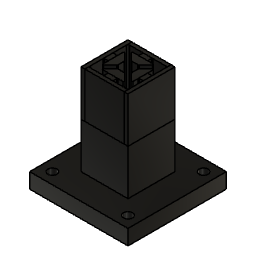
extrusion_hole (Autodesk Fusion 360 design; units mm, degrees)
Autodesk Fusion 360 part; units mm, degrees
note: some values were not read from the file. Chosen so that the rebuilt part matches the saved one: which bodies a step acts on.
sketch "Sketch1" plane through (0, 0, 0) normal (0, 0, 1) x (1, 0, 0)
  line L0 (15.5, -15.5) -> (-15.5, -15.5)
  line L1 (-15.5, -15.5) -> (-15.5, 15.5)
  line L2 (-15.5, 15.5) -> (15.5, 15.5)
  line L3 (15.5, 15.5) -> (15.5, -15.5)
  line L4 (15.5, -15.5) -> (-15.5, 15.5) construction
  line L5 (-15.5, -15.5) -> (15.5, 15.5) construction
  dimension "d11" = 31
  dimension "d12" = 31
  constraint horizontal L0
  constraint perpendicular L0 L1
  constraint parallel L0 L2
  constraint parallel L1 L3
  constraint coincident L4 origin
  constraint coincident L5 origin
  measures "d11" distance of L1.end L2.end
  measures "d12" distance of L0.end L1.end
extrude "Extrude1" add sketch "Sketch1" along normal blind 30 makes body 1
sketch "Sketch2" plane through (0, 0, 30) normal (0, 0, 1) x (-1, 0, 0)
  line L0 (-15.5, -15.5) -> (15.5, -15.5)
  line L1 (15.5, -15.5) -> (15.5, 15.5)
  line L2 (15.5, 15.5) -> (-15.5, 15.5)
  line L3 (-15.5, 15.5) -> (-15.5, -15.5)
  line L4 (-10.5, 3.5) -> (-12.5, 3.5)
  line L5 (10.5, 3.5) -> (10.5, 9.0858)
  line L6 (9.0858, -10.5) -> (2.5858, -4)
  line L7 (-12.5, -3.5) -> (-10.5, -3.5)
  line L8 (-10.5, 9.0858) -> (-10.5, 3.5)
  line L9 (9.0858, 10.5) -> (3.5, 10.5)
  line L10 (0, 0) -> (-4, 4) construction
  line L11 (-9.0858, -10.5) -> (-3.5, -10.5)
  line L12 (-9.0858, 10.5) -> (-2.5858, 4)
  line L13 (3.5, -12.5) -> (3.5, -10.5)
  line L14 (10.5, -3.5) -> (12.5, -3.5)
  line L15 (-2.5858, -4) -> (2.5858, -4)
  line L16 (-3.5, -10.5) -> (-3.5, -12.5)
  line L17 (2.5858, 4) -> (-2.5858, 4)
  line L18 (3.5, 10.5) -> (3.5, 12.5)
  line L19 (9.0858, 10.5) -> (2.5858, 4)
  line L20 (10.5, 9.0858) -> (4, 2.5858)
  line L21 (10.5, -9.0858) -> (4, -2.5858)
  line L22 (-10.5, -3.5) -> (-10.5, -9.0858)
  line L23 (-4, 2.5858) -> (-4, -2.5858)
  line L24 (3.5, -10.5) -> (9.0858, -10.5)
  line L25 (4, -2.5858) -> (4, 2.5858)
  line L26 (12.5, 3.5) -> (10.5, 3.5)
  line L27 (-3.5, -12.5) -> (-12.5, -12.5)
  line L28 (-12.5, 12.5) -> (-3.5, 12.5)
  line L29 (-10.5, -9.0858) -> (-4, -2.5858)
  line L30 (-9.0858, -10.5) -> (-2.5858, -4)
  line L31 (-3.5, 10.5) -> (-9.0858, 10.5)
  line L32 (-12.5, -12.5) -> (-12.5, -3.5)
  line L33 (12.5, -12.5) -> (3.5, -12.5)
  line L34 (10.5, -9.0858) -> (10.5, -3.5)
  line L35 (-12.5, 3.5) -> (-12.5, 12.5)
  line L36 (-3.5, 12.5) -> (-3.5, 10.5)
  line L37 (12.5, 12.5) -> (12.5, 3.5)
  line L38 (-10.5, 9.0858) -> (-4, 2.5858)
  line L39 (-4, -4) -> (0, 0) construction
  line L40 (3.5, 12.5) -> (12.5, 12.5)
  line L41 (12.5, -3.5) -> (12.5, -12.5)
  line L42 (10, 7.8787) -> (4.5, 2.3787)
  line L43 (4.5, -2.3787) -> (4.5, 2.3787)
  line L44 (10, -7.8787) -> (4.5, -2.3787)
  line L45 (10, -7.8787) -> (10, -3)
  line L46 (10, -3) -> (13, -3)
  line L47 (13, -3) -> (13, -13)
  line L48 (13, -13) -> (3, -13)
  line L49 (3, -13) -> (3, -10)
  line L50 (3, -10) -> (7.8787, -10)
  line L51 (7.8787, -10) -> (2.3787, -4.5)
  line L52 (-2.3787, -4.5) -> (2.3787, -4.5)
  line L53 (-7.8787, -10) -> (-2.3787, -4.5)
  line L54 (-7.8787, -10) -> (-3, -10)
  line L55 (-3, -10) -> (-3, -13)
  line L56 (-3, -13) -> (-13, -13)
  line L57 (-13, -13) -> (-13, -3)
  line L58 (-13, -3) -> (-10, -3)
  line L59 (-10, -3) -> (-10, -7.8787)
  line L60 (-10, -7.8787) -> (-4.5, -2.3787)
  line L61 (-4.5, 2.3787) -> (-4.5, -2.3787)
  line L62 (-10, 7.8787) -> (-4.5, 2.3787)
  line L63 (-10, 7.8787) -> (-10, 3)
  line L64 (-10, 3) -> (-13, 3)
  line L65 (-13, 3) -> (-13, 13)
  line L66 (-13, 13) -> (-3, 13)
  line L67 (-3, 13) -> (-3, 10)
  line L68 (-3, 10) -> (-7.8787, 10)
  line L69 (-7.8787, 10) -> (-2.3787, 4.5)
  line L70 (2.3787, 4.5) -> (-2.3787, 4.5)
  line L71 (7.8787, 10) -> (2.3787, 4.5)
  line L72 (7.8787, 10) -> (3, 10)
  line L73 (3, 10) -> (3, 13)
  line L74 (3, 13) -> (13, 13)
  line L75 (13, 13) -> (13, 3)
  line L76 (13, 3) -> (10, 3)
  line L77 (10, 3) -> (10, 7.8787)
  line L78 (4.5, -2.3787) -> (4.5, -4)
  line L79 (4.5, -4) -> (2.5858, -4)
  line L80 (4.5, -4) -> (5.3107, -3.1893)
  line L81 (10, -7.8787) -> (7.8787, -10)
  line L82 (10, -7.8787) -> (10, -10)
  line L83 (10, -10) -> (7.8787, -10)
  line L84 (4.5, -2.3787) -> (10, -2.3787)
  line L85 (10, -2.3787) -> (10, -7.8787)
  dimension "d16" = 360
  dimension "d17" = 8
  dimension "d18" = 2
  dimension "d19" = 2
  dimension "d20" = 2
  dimension "d21" = 9
  dimension "d22" = 9
  dimension "d23" = 135
  dimension "d24" = 8
  dimension "d25" = 0.5
  dimension "d32" = 9
  dimension "d33" = 9
  dimension "d34" = 1.1464
  dimension "d35" = 1.1464
  dimension "d36" = 2.1213
  dimension "d37" = 2.1213
  dimension "d38" = 3
  dimension "d39" = 4.7574
  dimension "d40" = 6
  dimension "d41" = 7.7782
  dimension "d42" = 5.5
  dimension "d43" = 5.5
  dimension "d44" = 5.5
  dimension "d45" = 10
  dimension "d46" = 12.5
  dimension "d47" = 2.5
  dimension "d48" = 31
  constraint horizontal L15
  constraint perpendicular L15 L25
  constraint parallel L15 L17
  constraint parallel L23 L25
  constraint coincident L10.start L39
  constraint coincident L39.end L10
  constraint coincident L10.start L39.end
  constraint perpendicular L13 L24
  constraint perpendicular L24 L34
  constraint parallel L6 L21
  constraint symmetric L6 L10 L21
  constraint perpendicular L15 L78
  constraint perpendicular L78 L79
  constraint coincident L44 L80.end
  constraint perpendicular L44 L80
  constraint perpendicular L51 L81
  constraint vertical L82
  constraint perpendicular L82 L83
  constraint perpendicular L45 L84
  constraint perpendicular L84 L85
  measures "d17" distance of L10.end L39.start
  measures "d18" distance of L6 L21
  measures "d19" distance of L14.start L14.end
  measures "d20" distance of L13.start L13.end
  measures "d21" distance of L13 L41
  measures "d22" distance of L14.end L33.start
  measures "d23" angle of L21 L25
  measures "d24" distance of L23 L25
  measures "d32" distance of L52 L70
  measures "d33" distance of L43 L61
  measures "d34" distance of L43.start L80
  measures "d35" distance of L78.end L80.end
  measures "d36" distance of L44.start L82.end
  measures "d37" distance of L50.end L82.end
  measures "d38" distance of L44.start L50.end
  measures "d39" distance of L42.end L43.start
  measures "d40" distance of L46 L76
  measures "d41" distance of L43.start L44.start
  measures "d42" distance of L43 L45.end
  measures "d43" distance of L44.start L84.end
  measures "d44" distance of L1 L85
  measures "d45" distance of L46 L48
  measures "d46" distance of L0 L46
  measures "d47" distance of L1 L47
  measures "d48" distance of L1 L3
extrude "Extrude2" add sketch "Sketch2" along normal blind 50 contours L0 L1 L2 L3 | L44 L45 L84 L85 bodies 1
fillet "Fillet1" radius 1 12 edges at (-13, 13, 55) (-4.5, 2.3787, 55) (-4.5, -2.3787, 55) (-13, -13, 55) (2.3787, -4.5, 55) (-2.3787, -4.5, 55) (-2.3787, 4.5, 55) (2.3787, 4.5, 55) (4.5, -2.3787, 55) (4.5, 2.3787, 55) (13, -13, 55) (13, 13, 55) on bodies 1
fillet "Fillet2" radius 0.5 24 edges at (-7.8787, 10, 55) (-10, 7.8787, 55) (-13, 3, 55) (-10, 3, 55) (-3, 10, 55) (-3, 13, 55) (3, 10, 55) (7.8787, 10, 55) (10, 7.8787, 55) (10, -7.8787, 55) (3, 13, 55) (10, 3, 55) (13, 3, 55) (10, -3, 55) (13, -3, 55) (7.8787, -10, 55) (3, -10, 55) (3, -13, 55) (-7.8787, -10, 55) (-10, -7.8787, 55) (-13, -3, 55) (-10, -3, 55) (-3, -10, 55) (-3, -13, 55) on bodies 1
extrude "Extrude3" cut 1 faces at (0.6548, 8.2857, 80) along direction (0, 0, -1) blind 20 on bodies 1 bodies 1
move_body "Move1" bodies 1 to x (1, 0, 0) y (0, 1, 0) z (0, 0, 1) at (0, 0, -30)
split "Split1" by plane through (0, 0, 0) normal (0, 0, 1) bodies 1 makes body 2 at (-15.5, -5.1667, 20)
split "Split2" by plane through (-13, 3, 0) normal (1, 0, 0) and through (13, 13, 0) normal (-1, 0, 0) bodies 2 makes body 3 at (-7.6953, -5.5739, 10) makes body 4 at (15.5, 5.1667, 20) makes body 5 at (4.3333, -15.5, 10) makes body 6 at (7.6953, 5.5739, 10) makes body 7 at (-4.3333, 15.5, 20)
split "Split3" by plane through (3, 13, 0) normal (0, -1, 0) and through (-3, 10, 0) normal (0, 1, 0) bodies 7 makes body 8 at (13, 12.3333, 10) makes body 9 at (-5.5739, 7.6953, 10) makes body 10 at (-12.9989, 12.0476, 10) makes body 11 at (3, 11.1667, 10)
split "Split4" by plane through (-3, -13, 0) normal (0, 1, 0) and through (3, -10, 0) normal (0, -1, 0) bodies 5 makes body 12 at (12.9989, -12.0476, 10) makes body 13 at (5.5739, -7.6953, 10) makes body 14 at (-13, -12.6667, 20) makes body 15 at (-3, -11.1667, 10)
split "Split5" by plane through (10, 3, 0) normal (1, 0, 0) bodies 6 makes body 16 at (13, 1.1667, 20)
split "Split6" by plane through (-10, -3, 0) normal (-1, 0, 0) bodies 3 makes body 17 at (-13, -1.1667, 20)
split "Split7" by plane through (3, 10, 0) normal (1, 0, 0) and through (-3, 13, 0) normal (-1, 0, 0) bodies 11 makes body 18 at (3.3333, 10, 10) makes body 19 at (3.4762, 12.9994, 10) makes body 20 at (-3.4762, 10.0006, 10) makes body 21 at (-3.0556, 12.7291, 10)
split "Split8" by plane through (-3, -10, 0) normal (-1, 0, 0) and through (3, -13, 0) normal (1, 0, 0) bodies 15 makes body 22 at (-3.4762, -10.0006, 10) makes body 23 at (-3.3333, -13, 10) makes body 24 at (3.0556, -10.2709, 10) makes body 25 at (3.4762, -12.9994, 10)
split "Split9" by plane through (10, -3, 0) normal (0, -1, 0) and through (13, 3, 0) normal (0, 1, 0) bodies 16 makes body 26 at (12.7291, -3.0556, 10) makes body 27 at (10.0006, -3.4762, 10) makes body 28 at (13, 3.1667, 10) makes body 29 at (10.2709, 3.0556, 10)
split "Split10" by plane through (-10, 3, 0) normal (0, 1, 0) and through (-13, -3, 0) normal (0, -1, 0) bodies 17 makes body 30 at (-10.2709, 3.0556, 10) makes body 31 at (-13, 3.1667, 20) makes body 32 at (-10.0006, -3.4762, 10) makes body 33 at (-12.7291, -3.0556, 10)
move_body "Move2" bodies 1 2 3 4 5 6 7 8 9 10 11 12 13 14 15 16 17 18 19 20 21 22 23 24 25 26 27 28 29 30 31 32 33 to x (1, 0, 0) y (0, 1, 0) z (0, 0, 1) at (0, 0, -30)
sketch "Sketch3" plane through (0, 0, -60) normal (0, 0, -1) x (1, 0, 0)
  line L0 (-15.5, -15.5) -> (15.5, -15.5)
  line L1 (15.5, -15.5) -> (15.5, 15.5)
  line L2 (15.5, 15.5) -> (-15.5, 15.5)
  line L3 (-15.5, 15.5) -> (-15.5, -15.5)
  line L4 (32.5, 32.5) -> (-32.5, 32.5)
  line L5 (-32.5, 32.5) -> (-32.5, -32.5)
  line L6 (-32.5, -32.5) -> (32.5, -32.5)
  line L7 (32.5, -32.5) -> (32.5, 32.5)
  line L8 (32.5, 32.5) -> (-32.5, -32.5) construction
  line L9 (-32.5, 32.5) -> (32.5, -32.5) construction
  circle A0 centre (25, 25) radius 3
  circle A1 centre (-25, 25) radius 3
  circle A2 centre (-25, -25) radius 3
  circle A3 centre (25, -25) radius 3
  dimension "d51" = 65
  dimension "d52" = 65
  dimension "d53" = 6
  dimension "d54" = 6
  dimension "d55" = 6
  dimension "d57" = 25
  dimension "d58" = 25
  dimension "d59" = 25
  dimension "d60" = 6
  dimension "d61" = 25
  constraint horizontal L4
  constraint perpendicular L4 L5
  constraint parallel L4 L6
  constraint parallel L5 L7
  constraint coincident L8 origin
  constraint coincident L9 origin
  constraint coincident L8 A0.centre
  constraint coincident L9 A1.centre
  constraint coincident L8 A2.centre
  constraint coincident L9 A3.centre
  measures "d51" distance of L4.start L4.end
  measures "d52" distance of L4.end L5.end
  measures "d53" diameter of A0
  measures "d54" diameter of A1
  measures "d55" diameter of A2
  measures "d57" horizontal distance of origin A0.centre
  measures "d58" horizontal distance of origin A1.centre
  measures "d59" horizontal distance of origin A2.centre
  measures "d60" diameter of A3
  measures "d61" horizontal distance of origin A3.centre
extrude "Extrude4" add sketch "Sketch3" along normal blind 10 contours L0 L1 L2 L3 | L4 L5 L6 L7 bodies 1
split "Split11" by plane through (0, 0, -60) normal (0, 0, 1) bodies 1 makes body 34 at (-5.1667, 5.1667, -30)
